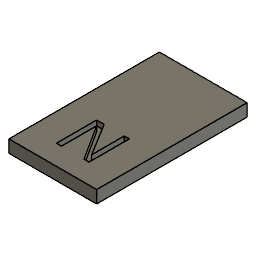
Tapa_N (Autodesk Fusion 360 design; units mm, degrees)
part number: 2025-11-07-13-48-39-675
Autodesk Fusion 360 part; units mm, degrees
note: some values were not read from the file. Set by a fixed rule: which sketch regions a step uses.
sketch "Boceto1" plane through (0, 0, 0) normal (0, 1, 0) x (1, 0, 0)
  line L0 (-50, 50) -> (-50, -10)
  line L1 (-50, 50) -> (-15, 50)
  line L2 (-15, 50) -> (-15, -10)
  line L3 (-15, -10) -> (-50, -10)
  dimension "d1" = 60
  dimension "d2" = 35
  constraint vertical L0
  constraint perpendicular L0 L1
  constraint perpendicular L1 L2
  constraint perpendicular L0 L3
  measures "d1" distance of L0.start L0.end
  measures "d2" distance of L0.start L1.end
extrude "Extruir1" add sketch "Boceto1" along normal blind 3
sketch "Boceto2" plane through (0, 0, 0) normal (0, -1, 0) x (1, 0, 0)
  line L0 (-50, 10) -> (-50, -50)
  line L1 (-50, -50) -> (-15, -50)
  line L2 (-15, -50) -> (-15, 10)
  line L3 (-15, 10) -> (-50, 10)
  line L4 (-36, -40) -> (-35, -24)
  line L5 (-29, -40) -> (-30, -24)
  arc A0 (-30, -24) -> (-35, -24) centre (-32.5, -24.0037) ccw
  arc A1 (-36, -40) -> (-29, -40) centre (-32.5, -39.997) ccw
  arc A2 (-36, -40) -> (-29, -40) centre (-32.5, -39.997) ccw
  constraint coincident A1.centre A2.centre
extrude "Extruir2" add 1 faces at (-38.3333, 3, -30) along direction (0, 1, 0) blind 2
extrude "Extruir3" cut sketch "Boceto2" against normal blind 2 contours L4 L5 A0 A1 A2
sketch "Boceto3" plane through (0, 5, 0) normal (0, 1, 0) x (-1, 0, 0)
  line L0 (50, -50) -> (50, 10)
  line L1 (50, 10) -> (15, 10)
  line L2 (15, 10) -> (15, -50)
  line L3 (15, -50) -> (50, -50)
  line L4 (39, -12) -> (39, 2)
  line L5 (39, 2) -> (37, 2)
  line L6 (37, 2) -> (37, -12)
  line L7 (50, 10) -> (32.5, 10)
  line L8 (28, 2) -> (26, 2)
  line L9 (26, 2) -> (26, -12)
  line L10 (39, -12) -> (39, -14)
  line L11 (39, -14) -> (37, -14)
  line L12 (28, -14) -> (26, -14)
  line L13 (26, -14) -> (26, -12)
  line L14 (37, -12) -> (28, 2)
  line L15 (28, -12) -> (28, -14)
  line L16 (37, -14) -> (36, -14)
  line L17 (36, -14) -> (28, -1)
  line L18 (28, -1) -> (28, -12)
  constraint parallel L0 L4
  constraint perpendicular L4 L5
  constraint perpendicular L5 L6
  constraint coincident L0.end L1.start
  constraint midpoint L1 L7.end
  constraint perpendicular L8 L9
  constraint parallel L4 L10
  constraint perpendicular L10 L11
  constraint parallel L11 L12
  constraint perpendicular L12 L13
  constraint perpendicular L12 L15
  constraint perpendicular L0 L16
  constraint perpendicular L16 L18
extrude "Extruir4" cut sketch "Boceto3" against normal blind 2 contours L4 L5 L6 L8 L9 L10 L11 L12 L13 L14 L15 L16 L17 L18
